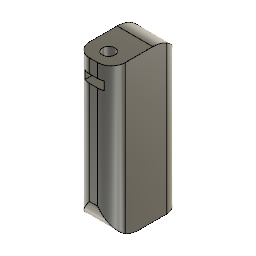
Bottom connector (Autodesk Fusion 360 design; units mm, degrees)
Autodesk Fusion 360 part; units mm, degrees
note: some values were not read from the file. Chosen so that the rebuilt part matches the saved one: which pieces of a blend or face edit are solid. Set by a fixed rule: which sketch regions a step uses.
sketch "Sketch2" plane through (0, 0, 0) normal (1, 0, 0) x (0, 1, 0)
  line L0 (0, 0) -> (25, 0)
  line L1 (25, 0) -> (25, 55)
  line L2 (25, 55) -> (0, 55)
  line L3 (0, 55) -> (0, 0)
  line L4 (12.5, 55) -> (12.5, 0) construction
  dimension "d5" = 25
  dimension "d6" = 55
  constraint horizontal L0
  constraint vertical L1
  constraint horizontal L2
  constraint vertical L3
  constraint coincident L0.start L3.end
  constraint midpoint L2 L4.start
  constraint midpoint L0 L4.end
  measures "d5" distance of L0.start L0.end
  measures "d6" distance of L0.start L2.end
extrude "Extrude2" add sketch "Sketch2" along normal blind 13
sketch "Sketch3" plane through (0, 0, 55) normal (0, 0, 1) x (-1, 0, 0)
  line L0 (0, -25) -> (0, 0)
  line L1 (0, 0) -> (-13, 0)
  line L2 (-13, 0) -> (-13, -25)
  line L3 (-13, -25) -> (0, -25)
  line L4 (-6.5, -25) -> (-6.5, 0) construction
  line L5 (-6.5, -12.5) -> (0, -12.5) construction
  circle A0 centre (-6.5, -19.5) radius 2.25
  circle A1 centre (-6.5, -5.5) radius 2.25
  line L6 (-10, -7.5207) -> (-6.5, -9.5415)
  line L7 (-6.5, -9.5415) -> (-3, -7.5207)
  line L8 (-3, -7.5207) -> (-3, -3.4793)
  line L9 (-3, -3.4793) -> (-6.5, -1.4585)
  line L10 (-6.5, -1.4585) -> (-10, -3.4793)
  line L11 (-10, -3.4793) -> (-10, -7.5207)
  line L12 (-10, -21.5207) -> (-6.5, -23.5415)
  line L13 (-6.5, -23.5415) -> (-3, -21.5207)
  line L14 (-3, -21.5207) -> (-3, -17.4793)
  line L15 (-3, -17.4793) -> (-6.5, -15.4585)
  line L16 (-6.5, -15.4585) -> (-10, -17.4793)
  line L17 (-10, -17.4793) -> (-10, -21.5207)
  line L18 (-3, -21.5207) -> (-3, -25)
  line L19 (-10, -21.5207) -> (-10, -25)
  line L20 (-10, -3.4793) -> (-10, 0)
  line L21 (-3, -3.4793) -> (-3, 0)
  point P0 (-6.5, -5.5)
  point P1 (-6.5, -19.5)
  dimension "d11" = 4.5
  dimension "d12" = 4.5
  dimension "d13" = 7
  dimension "d14" = 7
  dimension "d24" = 3.5
  dimension "d25" = 3.5
  constraint midpoint L3 L4.start
  constraint midpoint L1 L4.end
  constraint midpoint L0 L5.end
  constraint perpendicular L0 L5
  constraint coincident L4 P1
  constraint coincident L4 P0
  constraint coincident P0 A1.centre
  constraint coincident P1 A0.centre
  constraint coincident L3 L18.end
  constraint perpendicular L3 L18
  constraint coincident L3 L19.end
  constraint perpendicular L3 L19
  constraint coincident L1 L20.end
  constraint perpendicular L1 L20
  constraint coincident L1 L21.end
  constraint perpendicular L1 L21
  measures "d11" diameter of A0
  measures "d12" diameter of A1
  measures "d13" distance of L5.start P1
  measures "d14" distance of L5.start P0
  measures "d24" distance of P0 L11
  measures "d25" distance of P1 L17
extrude "Extrude3" cut sketch "Sketch3" against normal blind 25 contours A1
extrude "Extrude4" cut sketch "Sketch3" along normal blind 25 from surface at -55 contours A0
extrude "Extrude5" cut sketch "Sketch3" along normal blind 3.5 from surface at -50 contours L3 L12 L13 L18 L19 | L12 L13 L14 L15 L16 L17 | A0
extrude "Extrude6" cut sketch "Sketch3" against normal blind 3 from surface at -5 contours L1 L9 L10 L20 L21 | L6 L7 L8 L9 L10 L11
fillet "Fillet1" radius 5 4 edges at (0, 25, 27.5) (13, 25, 27.5) (13, 0, 27.5) (0, 0, 27.5)
fillet "Fillet1" radius 10 2 edges at (6.5, 25, 55) (6.5, 0, 0)
sketch "Sketch4" plane through (0, 25, 0) normal (0, 1, 0) x (-1, 0, 0)
  line L0 (-5, 8.5) -> (-5, 45)
  line L1 (-5, 45) -> (-8, 45)
  line L2 (-8, 45) -> (-8, 8.5)
  line L3 (-8, 8.5) -> (-5, 8.5)
  line L4 (-5, 0) -> (-5, 5) construction
  line L5 (-5, 5) -> (-8, 5) construction
  line L6 (-8, 5) -> (-8, 0) construction
  line L7 (-8, 0) -> (-5, 0) construction
  line L8 (-6.5, 0) -> (-6.5, 25) construction
  line L9 (-3, 26.75) -> (-10, 26.75)
  line L10 (-10, 26.75) -> (-10, 23.25)
  line L11 (-10, 23.25) -> (-3, 23.25)
  line L12 (-3, 23.25) -> (-3, 26.75)
  line L13 (-3, 26.75) -> (-10, 23.25) construction
  line L14 (-10, 26.75) -> (-3, 23.25) construction
  point P0 (-6.5, 25)
  dimension "d34" = 25
  dimension "d35" = 7
  dimension "d36" = 3.5
  constraint midpoint L7 L8.start
  constraint perpendicular L7 L8
  constraint perpendicular L9 L10
  constraint parallel L9 L11
  constraint parallel L10 L12
  constraint horizontal L9
  constraint coincident L13 P0
  constraint coincident L14 P0
  constraint coincident P0 L8.end
  measures "d34" distance of L8.start P0
  measures "d35" distance of L10.end L11.end
  measures "d36" distance of L9.end L10.end
extrude "Extrude7" [rolled back] along distance -9.5 taper angle 0
ref_plane "WorkPlane1" through (0, 0, 23) normal (0, 0, 1) x (1, 0, 0)
sketch "Sketch5" plane through (0, 0, 23) normal (0, 0, 1) x (1, 0, 0)
  line L0 (41.7693, 29.4739) -> (11.2693, 29.4739)
  line L1 (-15.2307, 32.4739) -> (-15.2307, 86.4739)
  line L2 (-12.2307, 89.4739) -> (41.7693, 89.4739)
  line L3 (44.7693, 86.4739) -> (44.7693, 32.4739)
  line L4 (39.7693, 34.4739) -> (-10.2307, 34.4739) construction
  line L5 (-10.2307, 34.4739) -> (-10.2307, 84.4739) construction
  line L6 (-10.2307, 84.4739) -> (39.7693, 84.4739) construction
  line L7 (39.7693, 84.4739) -> (39.7693, 34.4739) construction
  circle A0 centre (39.7693, 84.4739) radius 2.25
  circle A1 centre (-10.2307, 84.4739) radius 2.25
  circle A2 centre (-10.2307, 34.4739) radius 2.25
  circle A3 centre (39.7693, 34.4739) radius 2.25
  arc A4 (44.7693, 86.4739) -> (41.7693, 89.4739) centre (41.7693, 86.4739) ccw
  arc A5 (-12.2307, 89.4739) -> (-15.2307, 86.4739) centre (-12.2307, 86.4739) ccw
  arc A6 (-15.2307, 32.4739) -> (-12.2307, 29.4739) centre (-12.2307, 32.4739) ccw
  arc A7 (41.7693, 29.4739) -> (44.7693, 32.4739) centre (41.7693, 32.4739) ccw
  line L8 (14.7693, 89.4739) -> (14.7693, 59.4739) construction
  circle A8 centre (14.7693, 59.4739) radius 29
  line L9 (10.2693, 28.4739) -> (10.2693, 16.4739)
  line L10 (9.2693, 15.4739) -> (3.7693, 15.4739)
  line L11 (2.7693, 16.4739) -> (2.7693, 28.4739)
  arc A9 (11.2693, 29.4739) -> (10.2693, 28.4739) centre (11.2693, 28.4739) ccw
  line L12 (-12.2307, 29.4739) -> (1.7693, 29.4739)
  arc A10 (2.7693, 28.4739) -> (1.7693, 29.4739) centre (1.7693, 28.4739) ccw
  arc A11 (2.7693, 16.4739) -> (3.7693, 15.4739) centre (3.7693, 16.4739) ccw
  arc A12 (9.2693, 15.4739) -> (10.2693, 16.4739) centre (9.2693, 16.4739) ccw
  circle A13 centre (6.5193, 19.4739) radius 2.25
  point P0 (44.7693, 29.4739)
  point P1 (-15.2307, 29.4739)
  point P2 (44.7693, 89.4739)
  point P3 (2.7693, 29.4739)
  point P4 (2.7693, 15.4739)
  dimension "d40" = 60
  dimension "d41" = 60
  dimension "d43" = 4.5
  dimension "d44" = 4.5
  dimension "d45" = 4.5
  dimension "d46" = 4.5
  dimension "d47" = 3
  dimension "d48" = 50
  dimension "d49" = 50
  dimension "d50" = 58
  dimension "d52" = 14
  dimension "d53" = 18
  dimension "d54" = 1
  dimension "d55" = 1
  dimension "d56" = 4.5
  dimension "d58" = 3.75
  dimension "d59" = 7.5
  dimension "d60" = 5
  dimension "d61" = 5
  dimension "d62" = 30
  dimension "d63" = 50
  dimension "d64" = 50
  dimension "d70" = 4
  constraint horizontal L0
  constraint vertical L1
  constraint horizontal L2
  constraint vertical L3
  constraint coincident L6.end L7.start
  constraint coincident L5.end L6.start
  constraint coincident L4.end L5.start
  constraint coincident L4.start L7.end
  constraint coincident P2 L2
  constraint coincident P2 L3
  constraint tangent L2 A4
  constraint tangent L3 A4
  constraint tangent L1 A5
  constraint tangent L2 A5
  constraint equal A4 A5
  constraint coincident P1 L0
  constraint coincident P1 L1
  constraint tangent L0 A6
  constraint tangent L1 A6
  constraint equal A4 A6
  constraint coincident P0 L0
  constraint coincident P0 L3
  constraint tangent L0 A7
  constraint tangent L3 A7
  constraint equal A4 A7
  constraint midpoint L2 L8.start
  constraint perpendicular L2 L8
  constraint coincident L8.end A8.centre
  constraint vertical L9
  constraint horizontal L10
  constraint vertical L11
  constraint coincident L0 P3
  constraint parallel L0 L4
  constraint parallel L1 L5
  constraint parallel L2 L6
  constraint parallel L3 L7
  constraint coincident L0 A6.end
  constraint tangent L0 A9
  constraint tangent L9 A9
  constraint coincident P3 L11
  constraint coincident P3 L12
  constraint tangent L11 A10
  constraint tangent L12 A10
  constraint coincident P4 L10
  constraint coincident P4 L11
  constraint tangent L10 A11
  constraint tangent L11 A11
  constraint equal A10 A11
  constraint tangent L9 A12
  constraint tangent L10 A12
  constraint equal A10 A12
  measures "d40" distance of P0 P1
  measures "d41" distance of P0 P2
  measures "d43" diameter of A0
  measures "d44" diameter of A1
  measures "d45" diameter of A2
  measures "d46" diameter of A3
  measures "d47" radius of A4
  measures "d48" distance of L4 L6
  measures "d49" distance of L5 L7
  measures "d50" diameter of A8
  measures "d52" distance of P3 P4
  measures "d53" distance of L1 P3
  measures "d54" radius of A9
  measures "d55" radius of A10
  measures "d56" diameter of A13
  measures "d58" distance of L9 A13.centre
  measures "d59" distance of L9 L11
  measures "d60" distance of L1 L5
  measures "d61" distance of L0 L4
  measures "d62" distance of L8.start L8.end
  measures "d63" distance of L4.start L6.end
  measures "d64" distance of L4.start L4.end
  measures "d70" distance of L10 A13.centre
extrude "Extrude8" [rolled back] along distance 3 taper angle 0
extrude "Extrude9" [rolled back] along distance -25 taper angle 0
named bodies: "btm_connection", "fan_mount", "Noctua NF-A6x25"
